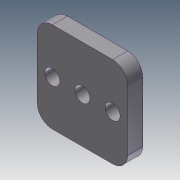
# Autodesk Inventor part: J005646
Saved by Autodesk Inventor 2015 SP1 (Build 190203100, 203)
## iProperties
Created: 2014-12-01
Material: Generic
Vendor: HHMI: JFRC - ID&F
Document SubType Name: Modeling
Designer: ARNOLDJ
Density: 1 g/cm^3
Appearance: Default
Description: SPACER FOR BALL CAMERA
Part Number: J005646
RuleStatus: InUse
AfterDocSave0: file://Part Number Cleaner
DESIGN DEPARTMENT: HHMI: JFRC - ID&F
ALTERED ITEM PART NUMBER: N/A
ALTERED ITEM VENDOR: N/A
ALTERED ITEM DESCRIPTION: N/A
Revision Number: 0
Autodesk Inventor part; units mm, degrees
ref_plane "YZ Plane" through (0, 0, 0) normal (1, 0, 0) x (0, 1, 0)
ref_plane "XZ Plane" through (0, 0, 0) normal (0, 1, 0) x (-1, 0, 0)
ref_plane "XY Plane" through (0, 0, 0) normal (0, 0, 1) x (1, 0, 0)
sketch "Sketch1" plane through (0, 0, 0) normal (0, 0, 1) x (1, 0, 0)
  line L0 (-19.05, 19.05) -> (19.05, 19.05)
  line L1 (19.05, 19.05) -> (19.05, -19.05)
  line L2 (19.05, -19.05) -> (-19.05, -19.05)
  line L3 (-19.05, -19.05) -> (-19.05, 19.05)
  line L4 (0, 19.05) -> (0, -19.05) construction
  line L5 (-19.05, 0) -> (19.05, 0) construction
  point P0 (0, 0)
  point P1 (0, 0)
  dimension "d0" = 38.1
  dimension "d1" = 38.1
  constraints: 12 end point, 5 midpoint, 2 parallel, 2 vertical alignment, 1 horizontal, 1 horizontal alignment, 1 perpendicular
  measures "d0" distance of L0.start L0.end
  measures "d1" distance of L2.end L0.start
extrude "Extrusion1" add sketch "Sketch1" along normal blind 6.35
sketch "Sketch2" plane through (0, 0, 0) normal (0, 0, 1) x (1, 0, 0)
  point P0 (0, 0)
  point P1 (0, 0)
  point P2 (-12.7, 0)
  point P3 (12.7, 0)
  dimension "d4" = 12.7
  dimension "d5" = 12.7
  constraints: 1 coincident
  measures "d4" distance of point (0, 0) point (-12.7, 0)
  measures "d5" distance of point (0, 0) point (12.7, 0)
hole "Hole1" at (0, 0, 0) at (-12.7, 0, 0) at (12.7, 0, 0) direction (0, 0, 1) diameter 6.35 end through all
fillet "Fillet1" radius 6.35 4 edges at (19.05, -19.05, 3.175) (19.05, 19.05, 3.175) (-19.05, 19.05, 3.175) (-19.05, -19.05, 3.175)
body "Solid1"
